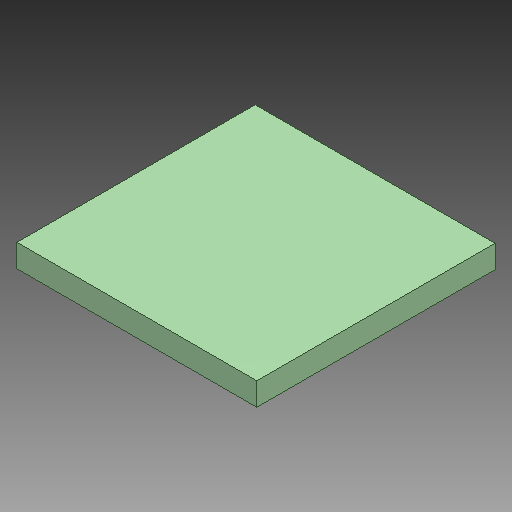
# Autodesk Inventor part: 3CTH
Saved by Autodesk Inventor 2017.3 (Build 213256000, 256)
## iProperties
Part Number: 3CTH
Material: Generisch
Document SubType Name: Modeling
Designer: Nils
Density: 1 g/cm^3
Appearance: 3CTH, 3CTH
Author: Nils
Autodesk Inventor part; units mm, degrees
ref_plane "YZ Plane" through (0, 0, 0) normal (1, 0, 0) x (0, 1, 0)
ref_plane "XZ Plane" through (0, 0, 0) normal (0, 1, 0) x (-1, 0, 0)
ref_plane "XY Plane" through (0, 0, 0) normal (0, 0, 1) x (1, 0, 0)
sketch "3CTH, 3CTH_41" plane through (0, 0, 0) normal (0, 0, 1) x (1, 0, 0)
  line L0 (-5.2428, 5.2) -> (5.2299, 5.2)
  line L1 (5.2299, 5.2) -> (5.2299, -5.2)
  line L2 (5.2299, -5.2) -> (-5.2428, -5.2)
  line L3 (-5.2428, -5.2) -> (-5.2428, 5.2)
  constraints: 8 end point
extrude "Extrusion1" add sketch "3CTH, 3CTH_41" along normal blind 1
